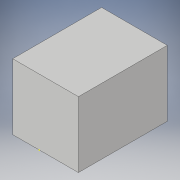
# Autodesk Inventor part: Part20
Saved by Autodesk Inventor 2019 (Build 230136000, 136)
## iProperties
Created: 2021-08-31
Part Number: Part20
Material: 一般
Document SubType Name: Sheet Metal
Designer: yuta
Density: 1 g/cm^3
Sheet Metal Rule: Default_mm
Appearance: 既定
Author: yuta
Autodesk Inventor part; units mm, degrees
ref_plane "YZ Plane" through (0, 0, 0) normal (1, 0, 0) x (0, 1, 0)
ref_plane "XZ Plane" through (0, 0, 0) normal (0, 1, 0) x (-1, 0, 0)
ref_plane "XY Plane" through (0, 0, 0) normal (0, 0, 1) x (1, 0, 0)
sketch "スケッチ1" plane through (0, 0, 0) normal (0, 1, 0) x (-1, 0, 0)
  line L0 (8.1505, 14.0302) -> (-11.8495, 14.0302)
  line L1 (-11.8495, 14.0302) -> (-11.8495, -13.0164)
  line L2 (-11.8495, -13.0164) -> (8.1505, -13.0164)
  line L3 (8.1505, -13.0164) -> (8.1505, 14.0302)
  point P0 (0, 0)
  dimension "d0" = 20
  constraints: 8 end point, 2 parallel, 1 horizontal, 1 perpendicular
  measures "d0" distance of L2.end L1.end
extrude "押し出し1" add sketch "スケッチ1" along normal blind 20
sketch "スケッチ2" plane through (-8.1505, 0, 14.0302) normal (0, 0, 1) x (1, 0, 0)
  point P0 (8.1505, 0)
sketch "スケッチ3" plane through (11.8495, 0, -13.0164) normal (0, 0, -1) x (-1, 0, 0)
  circle A0 centre (10, 10) radius 3
  line L0 (0, 20) -> (20, 20) projected
  line L1 (20, 0) -> (20, 20) projected
  point P0 (11.8495, 0)
  dimension "d3" = 6
  dimension "d4" = 10
  dimension "d5" = 10
  constraints: 1 centre point
  measures "d3" diameter of A0
  measures "d4" distance from line of L0 A0.centre
  measures "d5" distance from line of L1 A0.centre
hole "穴1" at (1.8495, 10, -13.0164) direction (0, 0, 1) diameter 6 depth 10
equation "\"BendRadius\" = Thickness"
equation "\"BendReliefWidth\" = Thickness"
equation "\"BendReliefDepth\" = 0.5 * Thickness"
equation "\"CornerReliefSize\" = 4 * Thickness"
equation "\"MinimumRemnant\" = 2 * Thickness"
equation "\"TransitionRadius\" = BendRadius"
equation "\"JacobiRadiusSize\" = BendRadius"
equation "\"GapSize\" = Thickness"
equation "\"Thickness\" = 0.5"
